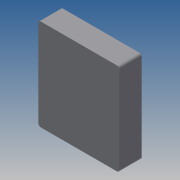
# Autodesk Inventor part: Insert
Saved by Autodesk Inventor 2014 (Build 180170000, 170)
## iProperties
Created: 2014-05-15
Part Number: Insert
Material: Generic
Document SubType Name: Modeling
Designer: 1770749
Density: 1 g/cm^3
Appearance: Default
Author: 1770749
Autodesk Inventor part; units mm, degrees
ref_plane "YZ Plane" through (0, 0, 0) normal (1, 0, 0) x (0, 1, 0)
ref_plane "XZ Plane" through (0, 0, 0) normal (0, 1, 0) x (-1, 0, 0)
ref_plane "XY Plane" through (0, 0, 0) normal (0, 0, 1) x (1, 0, 0)
sketch "Sketch1" plane through (0, 0, 0) normal (0, 1, 0) x (-1, 0, 0)
  line L0 (0, 0) -> (62, 0)
  line L1 (62, 0) -> (62, 70)
  line L2 (62, 70) -> (0, 70)
  line L3 (0, 70) -> (0, 0)
  dimension "d0" = 62
  dimension "d1" = 70
  constraints: 8 end point, 2 parallel, 1 horizontal, 1 perpendicular
  measures "d0" distance of L2.end L1.end
  measures "d1" distance of L1.end L0.end
extrude "Extrusion1" add sketch "Sketch1" along normal blind 2
sketch "Sketch2" plane through (0, 2, 0) normal (0, 1, 0) x (1, 0, 0)
  line L0 (0, 0) -> (-62, 0) projected
  line L1 (-62, 0) -> (-62, -70) projected
  line L2 (-62, -70) -> (0, -70) projected
  line L3 (0, -70) -> (0, 0) projected
  line L4 (-60, -2) -> (-2, -2)
  line L5 (-2, -2) -> (-2, -68)
  line L6 (-2, -68) -> (-60, -68)
  line L7 (-60, -68) -> (-60, -2)
  line L8 (0, 0) -> (-62, 0) projected
  line L9 (-62, 0) -> (-62, -70) projected
  line L10 (-62, -70) -> (0, -70) projected
  line L11 (0, -70) -> (0, 0) projected
  dimension "d4" = 2
  dimension "d5" = 2
  dimension "d6" = 2
  dimension "d7" = 2
  constraints: 8 end point, 2 parallel, 1 horizontal, 1 perpendicular
  measures "d4" distance between parallel lines of L0 L4
  measures "d5" distance between parallel lines of L1 L7
  measures "d6" distance between parallel lines of L2 L6
  measures "d7" distance between parallel lines of L3 L5
extrude "Extrusion2" add sketch "Sketch2" along normal blind 15
fillet "Fillet1" radius 2 4 edges at (-62, 8.5, 70) (-62, 8.5, 0) (0, 8.5, 0) (0, 8.5, 70)
body "Solid1"
